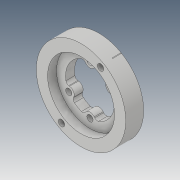
# Autodesk Inventor part: thrusterGimbalMount
Saved by Autodesk Inventor 2018 (Build 220112000, 112)
## iProperties
Created: 2020-01-09
Part Number: thrusterGimbalMount
Material: Generic
Document SubType Name: Modeling
Designer: anirudh
Density: 1 g/cm^3
Appearance: Default
Author: anirudh
Autodesk Inventor part; units mm, degrees
ref_plane "YZ Plane" through (0, 0, 0) normal (1, 0, 0) x (0, 1, 0)
ref_plane "XZ Plane" through (0, 0, 0) normal (0, 1, 0) x (-1, 0, 0)
ref_plane "XY Plane" through (0, 0, 0) normal (0, 0, 1) x (1, 0, 0)
sketch "Sketch1" plane through (0, 0, 0) normal (0, 0, 1) x (1, 0, 0)
  circle A0 centre (0, 0) radius 18.9992
  circle A1 centre (0, 13.8684) radius 1.75
  circle A2 centre (-12.010387, 6.9342) radius 1.75
  circle A3 centre (-12.010387, -6.9342) radius 1.75
  circle A4 centre (0, -13.8684) radius 1.75
  circle A5 centre (12.010387, -6.9342) radius 1.75
  circle A6 centre (12.010387, 6.9342) radius 1.75
  line L0 (0, 0) -> (12.883802, 0) construction
  arc A7 (-1.951996, 11.960156) -> (1.951996, 11.960156) centre (0, 12.1184) ccw
  arc A8 (-11.333797, 4.2896) -> (-9.381801, 7.670556) centre (-10.494842, 6.0592) ccw
  arc A9 (-1.951996, 11.960156) -> (-9.381801, 7.670556) centre (0, 0) ccw
  arc A10 (-9.381801, -7.670556) -> (-11.333797, -4.2896) centre (-10.494842, -6.0592) ccw
  arc A11 (-11.333797, 4.2896) -> (-11.333797, -4.2896) centre (0, 0) ccw
  arc A12 (1.951996, -11.960156) -> (-1.951996, -11.960156) centre (0, -12.1184) ccw
  arc A13 (-9.381801, -7.670556) -> (-1.951996, -11.960156) centre (0, 0) ccw
  arc A14 (1.951996, -11.960156) -> (9.381801, -7.670556) centre (0, 0) ccw
  arc A15 (11.333797, -4.2896) -> (9.381801, -7.670556) centre (10.494842, -6.0592) ccw
  arc A16 (11.333797, -4.2896) -> (11.333797, 4.2896) centre (0, 0) ccw
  arc A17 (9.381801, 7.670556) -> (1.951996, 11.960156) centre (0, 0) ccw
  arc A18 (9.381801, 7.670556) -> (11.333797, 4.2896) centre (10.494842, 6.0592) ccw
  dimension "d5" = 3.5
  dimension "d8" = 360
  constraints: 24 point on circle, 13 centre point, 2 coincident, 2 end point, 2 vertical alignment, 1 horizontal, 29 other
extrude "Extrusion1" add sketch "Sketch1" along normal blind 5.08
fillet "Fillet1" radius 1.905 12 edges at (-11.3338, 4.2896, 2.54) (-9.3818, 7.6706, 2.54) (-9.3818, -7.6706, 2.54) (-11.3338, -4.2896, 2.54) (-1.952, -11.9602, 2.54) (1.952, -11.9602, 2.54) (9.3818, -7.6706, 2.54) (11.3338, -4.2896, 2.54) (11.3338, 4.2896, 2.54) (9.3818, 7.6706, 2.54) (1.952, 11.9602, 2.54) (-1.952, 11.9602, 2.54)
sketch "Sketch2" plane through (0, 0, 5.08) normal (0, 0, 1) x (1, 0, 0)
  circle A0 centre (0, 0) radius 18.9992
  arc A1 (-22.1996, 3.2004) -> (-22.1996, -3.2004) centre (-22.1996, 0) ccw
  arc A2 (22.1996, -3.2004) -> (22.1996, 3.2004) centre (22.1996, 0) ccw
  circle A3 centre (-22.1996, 0) radius 1.8
  circle A4 centre (22.1996, 0) radius 1.8
  line L0 (-22.1996, -3.2004) -> (-18.727708, -3.2004)
  line L1 (-22.1996, 3.2004) -> (-18.727708, 3.2004)
  line L2 (22.1996, -3.2004) -> (18.727708, -3.2004)
  line L3 (22.1996, 3.2004) -> (18.727708, 3.2004)
  arc A5 (18.727708, -3.2004) -> (18.727708, 3.2004) centre (0, 0) ccw
  arc A6 (-18.727708, 3.2004) -> (-18.727708, -3.2004) centre (0, 0) ccw
  arc A7 (8.206333, 8.916934) -> (3.619125, 11.56536) centre (0, 0) ccw
  arc A8 (-12.135482, -14.618471) -> (-6.592226, -17.818871) centre (0, 0) ccw
  line L4 (-8.328172, -20.825618) -> (-6.592226, -17.818871)
  line L5 (-13.871428, -17.625218) -> (-12.135482, -14.618471)
  arc A9 (-13.871428, -17.625218) -> (-8.328172, -20.825618) centre (-11.0998, -19.225418) ccw
  circle A10 centre (-11.0998, -19.225418) radius 1.8
  arc A11 (12.135482, 14.618471) -> (6.592226, 17.818871) centre (0, 0) ccw
  line L6 (13.871428, 17.625218) -> (12.135482, 14.618471)
  line L7 (8.328172, 20.825618) -> (6.592226, 17.818871)
  circle A12 centre (11.0998, 19.225418) radius 1.8
  arc A13 (13.871428, 17.625218) -> (8.328172, 20.825618) centre (11.0998, 19.225418) ccw
  arc A14 (6.592226, -17.818871) -> (12.135482, -14.618471) centre (0, 0) ccw
  line L8 (13.871428, -17.625218) -> (12.135482, -14.618471)
  line L9 (8.328172, -20.825618) -> (6.592226, -17.818871)
  arc A15 (8.328172, -20.825618) -> (13.871428, -17.625218) centre (11.0998, -19.225418) ccw
  circle A16 centre (11.0998, -19.225418) radius 1.8
  arc A17 (-6.592226, 17.818871) -> (-12.135482, 14.618471) centre (0, 0) ccw
  line L10 (-8.328172, 20.825618) -> (-6.592226, 17.818871)
  line L11 (-13.871428, 17.625218) -> (-12.135482, 14.618471)
  circle A18 centre (-11.0998, 19.225418) radius 1.8
  arc A19 (-8.328172, 20.825618) -> (-13.871428, 17.625218) centre (-11.0998, 19.225418) ccw
  arc A20 (18.727708, -3.2004) -> (18.727708, 3.2004) centre (0, 0) ccw
  line L12 (22.1996, 3.2004) -> (18.727708, 3.2004)
  line L13 (22.1996, -3.2004) -> (18.727708, -3.2004)
  arc A21 (22.1996, -3.2004) -> (22.1996, 3.2004) centre (22.1996, 0) ccw
  circle A22 centre (22.1996, 0) radius 1.8
  arc A23 (-18.727708, 3.2004) -> (-18.727708, -3.2004) centre (0, 0) ccw
  line L14 (-22.1996, 3.2004) -> (-18.727708, 3.2004)
  line L15 (-22.1996, -3.2004) -> (-18.727708, -3.2004)
  circle A24 centre (-22.1996, 0) radius 1.8
  arc A25 (-22.1996, 3.2004) -> (-22.1996, -3.2004) centre (-22.1996, 0) ccw
  arc A26 (12.135482, 14.618471) -> (6.592226, 17.818871) centre (0, 0) ccw
  line L16 (8.328172, 20.825618) -> (6.592226, 17.818871)
  line L17 (13.871428, 17.625218) -> (12.135482, 14.618471)
  arc A27 (13.871428, 17.625218) -> (8.328172, 20.825618) centre (11.0998, 19.225418) ccw
  circle A28 centre (11.0998, 19.225418) radius 1.8
  arc A29 (-12.135482, -14.618471) -> (-6.592226, -17.818871) centre (0, 0) ccw
  line L18 (-13.871428, -17.625218) -> (-12.135482, -14.618471)
  line L19 (-8.328172, -20.825618) -> (-6.592226, -17.818871)
  circle A30 centre (-11.0998, -19.225418) radius 1.8
  arc A31 (-13.871428, -17.625218) -> (-8.328172, -20.825618) centre (-11.0998, -19.225418) ccw
  arc A32 (-6.592226, 17.818871) -> (-12.135482, 14.618471) centre (0, 0) ccw
  line L20 (-13.871428, 17.625218) -> (-12.135482, 14.618471)
  line L21 (-8.328172, 20.825618) -> (-6.592226, 17.818871)
  arc A33 (-8.328172, 20.825618) -> (-13.871428, 17.625218) centre (-11.0998, 19.225418) ccw
  circle A34 centre (-11.0998, 19.225418) radius 1.8
  arc A35 (6.592226, -17.818871) -> (12.135482, -14.618471) centre (0, 0) ccw
  line L22 (8.328172, -20.825618) -> (6.592226, -17.818871)
  line L23 (13.871428, -17.625218) -> (12.135482, -14.618471)
  circle A36 centre (11.0998, -19.225418) radius 1.8
  arc A37 (8.328172, -20.825618) -> (13.871428, -17.625218) centre (11.0998, -19.225418) ccw
  dimension "d30" = 360
  constraints: 48 end point, 48 point on circle, 36 centre point, 13 coincident, 4 horizontal, 139 other
sketch "Sketch4" plane through (0, 0, 5.08) normal (0, 0, 1) x (1, 0, 0)
  circle A0 centre (-12.010387, 6.9342) radius 1.75
  arc A1 (-1.546181, 10.916462) -> (-3.619125, 11.56536) centre (-3.050202, 9.747297) ccw
  arc A2 (-1.546181, 10.916462) -> (1.546181, 10.916462) centre (0, 12.1184) ccw
  line L0 (-1.546181, 10.916462) -> (-3.493287, 13.421232)
  arc A3 (3.619125, 11.56536) -> (1.546181, 10.916462) centre (3.050202, 9.747297) ccw
  line L1 (3.493287, 13.421232) -> (1.546181, 10.916462)
  arc A4 (-1.546181, 10.916462) -> (1.546181, 10.916462) centre (0, 12.1184) ccw
  line L2 (-10.227024, 4.119199) -> (-13.369771, 3.685341)
  arc A5 (-10.227024, 4.119199) -> (-8.680843, 6.797263) centre (-10.494842, 6.0592) ccw
  line L3 (-9.876484, 9.735891) -> (-8.680843, 6.797263)
  line L4 (-8.680843, -6.797263) -> (-9.876484, -9.735891)
  arc A6 (-8.680843, -6.797263) -> (-10.227024, -4.119199) centre (-10.494842, -6.0592) ccw
  line L5 (-13.369771, -3.685341) -> (-10.227024, -4.119199)
  line L6 (1.546181, -10.916462) -> (3.493287, -13.421232)
  arc A7 (1.546181, -10.916462) -> (-1.546181, -10.916462) centre (0, -12.1184) ccw
  line L7 (-3.493287, -13.421232) -> (-1.546181, -10.916462)
  line L8 (10.227024, -4.119199) -> (13.369771, -3.685341)
  arc A8 (10.227024, -4.119199) -> (8.680843, -6.797263) centre (10.494842, -6.0592) ccw
  line L9 (9.876484, -9.735891) -> (8.680843, -6.797263)
  line L10 (8.680843, 6.797263) -> (9.876484, 9.735891)
  arc A9 (8.680843, 6.797263) -> (10.227024, 4.119199) centre (10.494842, 6.0592) ccw
  line L11 (13.369771, 3.685341) -> (10.227024, 4.119199)
  arc A10 (-3.493287, 13.421232) -> (-9.876484, 9.735891) centre (0, 0) ccw
  arc A11 (-13.369771, 3.685341) -> (-13.369771, -3.685341) centre (0, 0) ccw
  arc A12 (-9.876484, -9.735891) -> (-3.493287, -13.421232) centre (0, 0) ccw
  arc A13 (3.493287, -13.421232) -> (9.876484, -9.735891) centre (0, 0) ccw
  arc A14 (13.369771, -3.685341) -> (13.369771, 3.685341) centre (0, 0) ccw
  arc A15 (9.876484, 9.735891) -> (3.493287, 13.421232) centre (0, 0) ccw
  dimension "d23" = 360
  constraints: 24 end point, 24 point on circle, 12 centre point, 2 coincident, 2 tangent, 49 other
extrude "Extrusion3" cut sketch "Sketch4" against normal blind 5.08 contours A2 L1 A15 L10 A9 L11 A14 L8 A8 L9 A13 L6 A7 L7 A12 L4 A6 L5 A11 L2 A5 L3 A10 L0
fillet "Fillet2" radius 1.905 12 edges at (-9.8765, 9.7359, 2.54) (-13.3698, 3.6853, 2.54) (-13.3698, -3.6853, 2.54) (-9.8765, -9.7359, 2.54) (-3.4933, -13.4212, 2.54) (3.4933, -13.4212, 2.54) (9.8765, -9.7359, 2.54) (13.3698, -3.6853, 2.54) (13.3698, 3.6853, 2.54) (9.8765, 9.7359, 2.54) (3.4933, 13.4212, 2.54) (-3.4933, 13.4212, 2.54)
extrude "Extrusion4" add sketch "Sketch2" against normal blind 5.08 contours A0 L7 A13 L6 | L4 A9 L5 A0
sketch "Sketch5" plane through (0, 0, 5.08) normal (0, 0, 1) x (1, 0, 0)
  circle A0 centre (-12.010387, 6.9342) radius 1.75
  arc A1 (-11.59569, 3.930254) -> (-9.201545, 8.077035) centre (-12.010387, 6.9342) ccw
  line L0 (-12.059066, 3.866285) -> (-10.227024, 4.119199)
  line L1 (-9.377833, 8.510315) -> (-8.680843, 6.797263)
  arc A2 (-10.227024, 4.119199) -> (-8.680843, 6.797263) centre (-10.494842, 6.0592) ccw
  line L2 (-11.59569, 3.930254) -> (-10.227024, 4.119199)
  line L3 (-9.201545, 8.077035) -> (-8.680843, 6.797263)
  arc A3 (-10.227024, 4.119199) -> (-8.680843, 6.797263) centre (-10.494842, 6.0592) ccw
  arc A4 (-9.201545, -8.077035) -> (-11.59569, -3.930254) centre (-12.010387, -6.9342) ccw
  line L4 (-9.201545, -8.077035) -> (-8.680843, -6.797263)
  line L5 (-11.59569, -3.930254) -> (-10.227024, -4.119199)
  arc A5 (-8.680843, -6.797263) -> (-10.227024, -4.119199) centre (-10.494842, -6.0592) ccw
  arc A6 (2.394145, -12.007289) -> (-2.394145, -12.007289) centre (0, -13.8684) ccw
  line L6 (2.394145, -12.007289) -> (1.546181, -10.916462)
  line L7 (-2.394145, -12.007289) -> (-1.546181, -10.916462)
  arc A7 (1.546181, -10.916462) -> (-1.546181, -10.916462) centre (0, -12.1184) ccw
  arc A8 (11.59569, -3.930254) -> (9.201545, -8.077035) centre (12.010387, -6.9342) ccw
  line L8 (11.59569, -3.930254) -> (10.227024, -4.119199)
  line L9 (9.201545, -8.077035) -> (8.680843, -6.797263)
  arc A9 (10.227024, -4.119199) -> (8.680843, -6.797263) centre (10.494842, -6.0592) ccw
  arc A10 (9.201545, 8.077035) -> (11.59569, 3.930254) centre (12.010387, 6.9342) ccw
  line L10 (9.201545, 8.077035) -> (8.680843, 6.797263)
  line L11 (11.59569, 3.930254) -> (10.227024, 4.119199)
  arc A11 (8.680843, 6.797263) -> (10.227024, 4.119199) centre (10.494842, 6.0592) ccw
  arc A12 (-2.394145, 12.007289) -> (2.394145, 12.007289) centre (0, 13.8684) ccw
  line L12 (-2.394145, 12.007289) -> (-1.546181, 10.916462)
  line L13 (2.394145, 12.007289) -> (1.546181, 10.916462)
  arc A13 (-1.546181, 10.916462) -> (1.546181, 10.916462) centre (0, 12.1184) ccw
  point P0 (0, 0)
  dimension "d36" = 360
  constraints: 25 end point, 24 point on circle, 12 centre point, 6 tangent, 2 coincident, 2 collinear, 2 point on line, 61 other
extrude "Extrusion5" cut sketch "Sketch5" against normal blind 5.08 contours A1 L1 A2 L0 | A4 L5 A5 L4 | A6 L7 A7 L6 | A8 L9 A9 L8 | A10 L11 A11 L10 | A12 L13 A13 L12
sketch "Sketch6" plane through (0, 0, 5.08) normal (0, 0, 1) x (1, 0, 0)
  arc A0 (-4.851695, 12.992058) -> (-8.825605, 10.69772) centre (0, 0) ccw
  arc A1 (-12.059066, 3.866285) -> (-13.6773, 2.294338) centre (-11.79855, 1.979182) ccw
  arc A2 (-12.059066, 3.866285) -> (-13.6773, 2.294338) centre (-11.79855, 1.979182) ccw
  arc A3 (-11.59569, 3.930254) -> (-9.201545, 8.077035) centre (-12.010387, 6.9342) ccw
  arc A4 (-8.825605, 10.69772) -> (-9.377833, 8.510315) centre (-7.613297, 9.228253) ccw
  arc A5 (-8.825605, 10.69772) -> (-9.377833, 8.510315) centre (-7.613297, 9.228253) ccw
  line L0 (-11.59569, 3.930254) -> (-12.059066, 3.866285)
  line L1 (-12.059066, 3.866285) -> (-11.59569, 3.930254)
  line L2 (-9.377833, 8.510315) -> (-9.201545, 8.077035)
  line L3 (-9.377833, 8.510315) -> (-9.201545, 8.077035)
  arc A6 (-11.59569, 3.930254) -> (-9.201545, 8.077035) centre (-12.010387, 6.9342) ccw
  arc A7 (8.825605, -10.69772) -> (9.377833, -8.510315) centre (7.613297, -9.228253) ccw
  arc A8 (8.825605, -10.69772) -> (9.377833, -8.510315) centre (7.613297, -9.228253) ccw
  arc A9 (11.59569, -3.930254) -> (9.201545, -8.077035) centre (12.010387, -6.9342) ccw
  arc A10 (12.059066, -3.866285) -> (13.6773, -2.294338) centre (11.79855, -1.979182) ccw
  arc A11 (12.059066, -3.866285) -> (13.6773, -2.294338) centre (11.79855, -1.979182) ccw
  line L4 (11.59569, -3.930254) -> (12.059066, -3.866285)
  line L5 (11.59569, -3.930254) -> (12.059066, -3.866285)
  line L6 (9.377833, -8.510315) -> (9.201545, -8.077035)
  line L7 (9.201545, -8.077035) -> (9.377833, -8.510315)
  arc A12 (11.59569, -3.930254) -> (9.201545, -8.077035) centre (12.010387, -6.9342) ccw
  arc A13 (-11.04151, 8.391519) -> (-12.788023, 5.366469) centre (-12.010387, 6.9342) ccw
  arc A14 (11.04151, -8.391519) -> (12.788023, -5.366469) centre (12.010387, -6.9342) ccw
  arc A15 (12.788023, -5.366469) -> (-11.04151, 8.391519) centre (0, 0) ccw
  arc A16 (-12.788023, 5.366469) -> (11.04151, -8.391519) centre (0, 0) ccw
  constraints: 24 point on circle, 12 tangent, 10 centre point, 9 coincident, 8 end point, 4 collinear
extrude "Extrusion6" cut sketch "Sketch6" against normal blind 5.08 contours A4 L2 A3 L0 A1 A16 A13 A15 | A15 A14 A16 A7 L6 A9 L4 A10
sketch "Sketch7" plane through (0, 0, 5.08) normal (0, 0, 1) x (1, 0, 0)
  arc A0 (-11.04151, 8.391519) -> (-12.788023, 5.366469) centre (-12.010387, 6.9342) ccw
  arc A1 (-11.04151, 8.391519) -> (-12.788023, 5.366469) centre (-12.010387, 6.9342) ccw
  arc A2 (11.04151, -8.391519) -> (12.788023, -5.366469) centre (12.010387, -6.9342) ccw
  arc A3 (11.04151, -8.391519) -> (12.788023, -5.366469) centre (12.010387, -6.9342) ccw
  circle A4 centre (0, 0) radius 13.8684
  constraints: 11 point on circle, 3 centre point, 3 coincident
extrude "Extrusion7" add sketch "Sketch7" against normal blind 5.08 contours A4 A0 | A4 A2
sketch "Sketch8" plane through (0, 0, 5.08) normal (0, 0, 1) x (1, 0, 0)
  circle A0 centre (0, 0) radius 25.395965
  line L0 (-12.135482, -14.618471) -> (-13.871428, -17.625218)
  circle A1 centre (0, 0) radius 18.9992
  circle A2 centre (-11.0998, -19.225418) radius 1.8
  circle A3 centre (11.0998, 19.225418) radius 1.8
  circle A4 centre (11.0998, 19.225418) radius 1.8
  constraints: 3 centre point, 3 coincident, 3 other
extrude "Extrusion8" add sketch "Sketch8" along normal blind 5.08 and the other way blind 5.08
body "Solid1"
